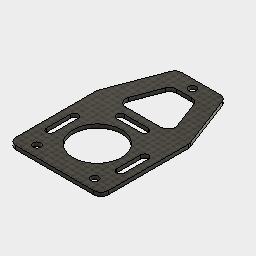
Camera Assembly (Autodesk Fusion 360 archive; units mm, degrees)
design "Camera Mounting Plate"
Autodesk Fusion 360 part; units mm, degrees
sketch "Sketch1" plane through (0, 0, 0) normal (0, 1, 0) x (1, 0, 0)
  circle A0 centre (-12, 0) radius 1.55
  circle A1 centre (12, 0) radius 1.55
  circle A2 centre (0, 13) radius 10
  line L0 (16.1, 13) -> (16.1, 18)
  line L1 (16.1, 13) -> (16.1, 8)
  line L2 (-16.1, 13) -> (-16.1, 18)
  line L3 (-16.1, 13) -> (-16.1, 8)
  line L4 (-13, 13) -> (-13, 18)
  line L5 (-13, 18) -> (-13, 13)
  line L6 (-13, 13) -> (-13, 8)
  line L7 (13, 13) -> (13, 18)
  line L8 (13, 13) -> (13, 8)
  arc A3 (-13, 18) -> (-16.1, 18) centre (-14.55, 18) ccw
  arc A4 (-16.1, 8) -> (-13, 8) centre (-14.55, 8) ccw
  arc A5 (16.1, 18) -> (13, 18) centre (14.55, 18) ccw
  arc A6 (13, 8) -> (16.1, 8) centre (14.55, 8) ccw
  line L9 (0, 29.1) -> (5, 29.1)
  line L10 (0, 29.1) -> (-5, 29.1)
  line L11 (0, 26) -> (5, 26)
  line L12 (5, 26) -> (0, 26)
  line L13 (0, 26) -> (-5, 26)
  arc A7 (-5, 29.1) -> (-5, 26) centre (-5, 27.55) ccw
  arc A8 (5, 26) -> (5, 29.1) centre (5, 27.55) ccw
  line L14 (12, -4.55) -> (16.1, -4.55)
  line L15 (19.1, -1.55) -> (19.1, 13)
  line L16 (-19.1, 13) -> (-19.1, -1.55)
  line L17 (-16.1, -4.55) -> (12, -4.55)
  arc A9 (16.1, -4.55) -> (19.1, -1.55) centre (16.1, -1.55) ccw
  arc A10 (-19.1, -1.55) -> (-16.1, -4.55) centre (-16.1, -1.55) ccw
  circle A11 centre (0, 52.45) radius 1.55
  line L18 (0, 55.95) -> (-7.9306, 55.95)
  line L19 (-19.1, 13) -> (-19.1, 31.4493)
  line L20 (19.1, 13) -> (19.1, 31.4493)
  line L21 (0, 55.95) -> (7.9306, 55.95)
  line L22 (10.735, 54.0156) -> (18.9044, 32.5148)
  line L23 (-10.735, 54.0156) -> (-18.9044, 32.5148)
  line L24 (0, 48.95) -> (3.1021, 48.95)
  line L25 (0, 48.95) -> (-3.1021, 48.95)
  line L26 (7.2626, 32) -> (-7.2626, 32)
  line L27 (10.067, 36.0656) -> (5.9065, 47.0156)
  line L28 (-10.067, 36.0656) -> (-5.9065, 47.0156)
  arc A12 (-10.067, 36.0656) -> (-7.2626, 32) centre (-7.2626, 35) ccw
  arc A13 (7.2626, 32) -> (10.067, 36.0656) centre (7.2626, 35) ccw
  arc A14 (5.9065, 47.0156) -> (3.1021, 48.95) centre (3.1021, 45.95) ccw
  arc A15 (-3.1021, 48.95) -> (-5.9065, 47.0156) centre (-3.1021, 45.95) ccw
  arc A16 (-18.9044, 32.5148) -> (-19.1, 31.4493) centre (-16.1, 31.4493) ccw
  arc A17 (19.1, 31.4493) -> (18.9044, 32.5148) centre (16.1, 31.4493) ccw
  arc A18 (10.735, 54.0156) -> (7.9306, 55.95) centre (7.9306, 52.95) ccw
  arc A19 (-7.9306, 55.95) -> (-10.735, 54.0156) centre (-7.9306, 52.95) ccw
  point P0 (-10, 55.95)
  point P1 (10, 55.95)
extrude "Extrude1" add sketch "Sketch1" along normal blind 1.5

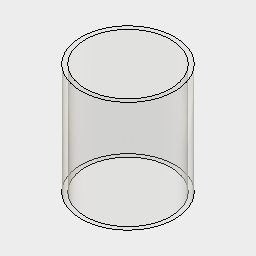
design "Acryllic Tube"
Autodesk Fusion 360 part; units mm, degrees
sketch "Sketch1" plane through (0, 0, 0) normal (0, 1, 0) x (1, 0, 0)
  circle A0 centre (0, 0) radius 27.5
  circle A1 centre (0, 0) radius 25
  dimension "d1" = 55
  measures "d1" diameter of A0
extrude "Extrude1" add sketch "Sketch1" along normal blind 65

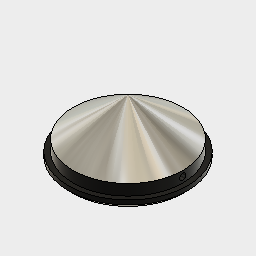
design "Camera Cap"
Autodesk Fusion 360 part; units mm, degrees
sketch "Sketch1" plane through (0, 0, 0) normal (0, 1, 0) x (1, 0, 0)
  circle A0 centre (0, 0) radius 27.5
  dimension "d1" = 55
  measures "d1" diameter of A0
extrude "Extrude1" add sketch "Sketch1" along normal blind 4
sketch "Sketch2" plane through (0, 4, 0) normal (0, 1, 0) x (-1, 0, 0)
  circle A0 centre (0, 0) radius 27.5
  circle A1 centre (0, 0) radius 25.3
  dimension "d4" = 50.6
  measures "d4" diameter of A1
extrude "Extrude2" add sketch "Sketch2" along normal blind 5 contours A1
sketch "Sketch3" plane through (0, 0, 0) normal (0, -1, 0) x (1, 0, 0)
  circle A0 centre (0, 0) radius 27.5
  line L0 (21.5985, 0) -> (19.1914, -4.1689)
  line L1 (3.5784, -14.5357) -> (-13.1761, -14.5877)
  line L2 (-11.9706, 0) -> (-14.3773, 4.1693)
  line L3 (-14.3773, 4.1693) -> (-5.9851, -10.3664)
  line L4 (14.3777, -4.1689) -> (6.0451, -18.7046)
  line L5 (5.9851, -10.3664) -> (3.5784, -14.5357)
  line L6 (-14.3773, 4.1693) -> (-6.0451, 18.705)
  line L7 (-5.9851, 18.705) -> (-14.3773, 4.1693)
  line L8 (-10.7992, -10.3664) -> (-19.2216, 4.1173)
  line L9 (-19.1914, 4.1693) -> (-10.7992, -10.3664)
  line L10 (-10.7992, -18.7046) -> (-13.2063, -14.5357)
  line L11 (-5.9851, -10.3664) -> (-10.7992, -10.3664)
  line L12 (-21.5985, 0) -> (-19.1914, 4.1693)
  line L13 (10.7992, 10.3668) -> (19.2216, -4.1169)
  line L14 (-10.7992, -10.3664) -> (5.9851, -10.3664)
  line L15 (-13.2063, -14.5357) -> (3.5784, -14.5357)
  line L16 (14.3777, -4.1689) -> (5.9851, 10.3668)
  line L17 (13.2063, 14.5357) -> (-3.578, 14.5357)
  line L18 (6.0451, -18.7046) -> (-10.7992, -18.7046)
  line L19 (11.9706, 0) -> (14.3777, -4.1689)
  line L20 (19.1914, -4.1689) -> (10.7992, 10.3668)
  line L21 (5.9851, -18.7046) -> (14.3777, -4.1689)
  line L22 (13.1765, 14.5877) -> (21.5985, 0)
  line L23 (-6.0451, 18.705) -> (10.7992, 18.705)
  line L24 (-3.578, 14.5357) -> (-11.9706, 0)
  line L25 (10.7992, 10.3668) -> (-5.9851, 10.3668)
  line L26 (10.7992, -18.7046) -> (5.9851, -18.7046)
  line L27 (19.2216, -4.1169) -> (10.7992, -18.7046)
  line L28 (10.7992, 18.705) -> (13.2063, 14.5357)
  line L29 (-11.9706, 0) -> (11.9706, 0)
  line L30 (0, 0) -> (0, 10.3668)
  line L31 (-19.2216, 4.1173) -> (-10.7992, 18.705)
  line L32 (-13.1761, -14.5877) -> (-21.5985, 0)
  line L33 (-10.7992, 18.705) -> (-5.9851, 18.705)
  line L34 (3.5784, -14.5357) -> (11.9706, 0)
  line L35 (5.9851, 10.3668) -> (10.7992, 10.3668)
  line L36 (-3.578, 14.5357) -> (13.1765, 14.5877)
  line L37 (-5.9851, 10.3668) -> (-3.578, 14.5357)
  line L38 (-13.2236, 4.171) -> (-5.4656, 17.705)
  line L39 (-5.4656, 17.705) -> (10.2219, 17.705)
  line L40 (10.2219, 17.705) -> (11.4743, 15.5357)
  line L41 (11.4743, 15.5357) -> (-4.1554, 15.5357)
  line L42 (-4.1554, 15.5357) -> (-11.9705, 2.0001)
  line L43 (-11.9705, 2.0001) -> (-13.2236, 4.171)
  line L44 (11.3766, 11.3668) -> (-4.253, 11.3668)
  line L45 (-4.253, 11.3668) -> (-2.9997, 13.5375)
  line L46 (-2.9997, 13.5375) -> (12.6002, 13.5859)
  line L47 (12.6002, 13.5859) -> (20.4438, 0)
  line L48 (20.4438, 0) -> (19.1914, -2.1689)
  line L49 (19.1914, -2.1689) -> (11.3766, 11.3668)
  line L50 (10.224, 9.3668) -> (18.0659, -4.1187)
  line L51 (18.0659, -4.1187) -> (10.2219, -17.7046)
  line L52 (10.2219, -17.7046) -> (7.7172, -17.7046)
  line L53 (7.7172, -17.7046) -> (15.5324, -4.1689)
  line L54 (15.5324, -4.1689) -> (7.7172, 9.3668)
  line L55 (7.7172, 9.3668) -> (10.224, 9.3668)
  line L56 (13.224, -4.1707) -> (5.4657, -17.7046)
  line L57 (5.4657, -17.7046) -> (-10.2219, -17.7046)
  line L58 (-10.2219, -17.7046) -> (-11.4742, -15.5357)
  line L59 (-11.4742, -15.5357) -> (4.1558, -15.5357)
  line L60 (4.1558, -15.5357) -> (11.9706, -2)
  line L61 (11.9706, -2) -> (13.224, -4.1707)
  line L62 (3, -13.5375) -> (-12.5998, -13.5859)
  line L63 (-12.5998, -13.5859) -> (-20.4438, 0)
  line L64 (-20.4438, 0) -> (-19.1914, 2.1693)
  line L65 (-19.1914, 2.1693) -> (-11.3766, -11.3664)
  line L66 (-11.3766, -11.3664) -> (4.2532, -11.3664)
  line L67 (4.2532, -11.3664) -> (3, -13.5375)
  line L68 (-10.224, -9.3664) -> (-18.0659, 4.1191)
  line L69 (-18.0659, 4.1191) -> (-10.2219, 17.705)
  line L70 (-10.2219, 17.705) -> (-7.7172, 17.705)
  line L71 (-7.7172, 17.705) -> (-15.532, 4.1693)
  line L72 (-15.532, 4.1693) -> (-7.7172, -9.3664)
  line L73 (-7.7172, -9.3664) -> (-10.224, -9.3664)
  dimension "d8" = 1
  dimension "d9" = 1
  dimension "d10" = 1
  dimension "d11" = 1
  dimension "d12" = 1
  dimension "d13" = 1
extrude "Extrude3" cut sketch "Sketch3" against normal blind 1 contours L38 L39 L40 L41 L42 L43 | L44 L45 L46 L47 L48 L49 | L50 L51 L52 L53 L54 L55 | L56 L57 L58 L59 L60 L61 | L62 L63 L64 L65 L66 L67 | L68 L69 L70 L71 L72 L73
chamfer "Chamfer1" distance 2 angle 45 1 edges at (-25.639, 0, 9.9444)
sketch "Sketch5" plane through (0, 0, 0) normal (0, 0, 1) x (1, 0, 0)
  line L0 (25.3, 9) -> (-25.3, 9)
  line L1 (25.3, 9) -> (0, 26.7153)
  line L2 (25.3, 9) -> (54.9449, 9) construction
  line L3 (0, 26.7153) -> (0, 9)
  line L4 (0, 26.7153) -> (0, 24.5)
  dimension "d19" = 145
  dimension "d37" = 30.8856
  measures "d19" angle of L1 L2
  measures "d37" distance of L0.start L1.end
revolve "Revolve1" add sketch "Sketch5" angle 360 about axis through (0, 1.75, 0) along (0, 1, 0)
ref_plane "WorkPlane3" through (25.3, 0, 0) normal (1, 0, 0) x (0, 1, 0)
sketch "Sketch8" plane through (25.3, 0, 0) normal (1, 0, 0) x (0, 0, -1)
  line L0 (0, 9) -> (0, 6.5)
  circle A0 centre (0, 6.5) radius 1.4
  point P0 (0, 9)
  dimension "d28" = 2.5
  dimension "d29" = 2.8
  measures "d28" distance of P0 L0.end
  measures "d29" diameter of A0
extrude "Extrude6" cut sketch "Sketch8" against normal blind 8
ref_plane "WorkPlane4" through (-25.3, 0, 0) normal (1, 0, 0) x (0, 1, 0)
sketch "Sketch9" plane through (-25.3, 0, 0) normal (1, 0, 0) x (0, 0, -1)
  line L0 (0, 9) -> (0, 6.5)
  circle A0 centre (0, 6.5) radius 1.4
  point P0 (0, 9)
  dimension "d33" = 2.5
  dimension "d34" = 2.8
  measures "d33" distance of P0 L0.end
  measures "d34" diameter of A0
extrude "Extrude7" cut sketch "Sketch9" along normal blind 8

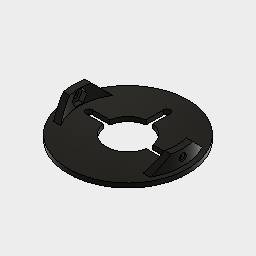
design "Camera Tube Mount"
Autodesk Fusion 360 part; units mm, degrees
sketch "Sketch1" plane through (0, 0, 0) normal (0, 1, 0) x (1, 0, 0)
  circle A0 centre (0, 0) radius 27.5
  circle A1 centre (0, 0) radius 10
  line L0 (0, 0) -> (13, 0)
  line L1 (0, 0) -> (0, 13)
  line L2 (0, 0) -> (-13, 0)
  line L3 (-13, 0) -> (-13, 1.55)
  line L4 (-13, 1.55) -> (-18, 1.55)
  line L5 (-13, 1.55) -> (-9.8791, 1.55)
  line L6 (-13, 0) -> (-13, -1.55)
  line L7 (-13, -1.55) -> (-9.8791, -1.55)
  line L8 (-13, -1.55) -> (-18, -1.55)
  line L9 (0, 13) -> (1.55, 13)
  line L10 (1.55, 13) -> (1.55, 18)
  line L11 (1.55, 18) -> (-1.55, 18)
  line L12 (-1.55, 18) -> (-1.55, 9.8791)
  line L13 (1.55, 9.8791) -> (1.55, 18)
  line L14 (13, 0) -> (13, -1.55)
  line L15 (13, -1.55) -> (18, -1.55)
  line L16 (18, -1.55) -> (9.8791, -1.55)
  line L17 (9.8791, 1.55) -> (18, 1.55)
  line L18 (18, 1.55) -> (18, -1.55)
  arc A2 (-18, 1.55) -> (-18, -1.55) centre (-18, 0) ccw
  arc A3 (1.55, 18) -> (-1.55, 18) centre (0, 18) ccw
  arc A4 (18, -1.55) -> (18, 1.55) centre (18, 0) ccw
  dimension "d12" = 13
  dimension "d13" = 13
  dimension "d14" = 13
  dimension "d15" = 1.55
  dimension "d16" = 5
  dimension "d17" = 1.55
  dimension "d18" = 1.55
  dimension "d19" = 5
  dimension "d20" = 3.1
  dimension "d21" = 1.55
  dimension "d22" = 5
  dimension "d23" = 3.1
  measures "d12" distance of A0.centre L0.end
  measures "d13" distance of A0.centre L1.end
  measures "d14" distance of A0.centre L2.end
  measures "d15" distance of L2.end L3.end
  measures "d16" distance of L3.end L4.end
  measures "d17" distance of L2.end L6.end
  measures "d18" distance of L1.end L9.end
  measures "d19" distance of L9.end L10.end
  measures "d20" distance of L10.end L11.end
  measures "d21" distance of L0.end L14.end
  measures "d22" distance of L14.end L15.end
  measures "d23" distance of L15.end L17.end
extrude "Extrude1" add sketch "Sketch1" along normal blind 2
sketch "Sketch2" plane through (0, 2, 0) normal (0, 1, 0) x (-1, 0, 0)
  line L0 (-18, 1.55) -> (-9.8791, 1.55)
  arc A0 (9.8791, 1.55) -> (-9.8791, 1.55) centre (0, 0) ccw
  line L1 (9.8791, 1.55) -> (18, 1.55)
  arc A1 (18, -1.55) -> (18, 1.55) centre (18, 0) ccw
  line L2 (18, -1.55) -> (9.8791, -1.55)
  arc A2 (1.55, -9.8791) -> (9.8791, -1.55) centre (0, 0) ccw
  line L3 (1.55, -9.8791) -> (1.55, -18)
  arc A3 (-1.55, -18) -> (1.55, -18) centre (0, -18) ccw
  line L4 (-1.55, -18) -> (-1.55, -9.8791)
  arc A4 (-9.8791, -1.55) -> (-1.55, -9.8791) centre (0, 0) ccw
  line L5 (-9.8791, -1.55) -> (-18, -1.55)
  arc A5 (-18, 1.55) -> (-18, -1.55) centre (-18, 0) ccw
  circle A6 centre (0, 0) radius 27.5
  circle A7 centre (0, 0) radius 25.3
  circle A8 centre (0, 0) radius 22.5
  dimension "d26" = 50.6
  dimension "d27" = 45
  measures "d26" diameter of A7
  measures "d27" diameter of A8
extrude "Extrude2" add sketch "Sketch2" along normal blind 7 contours A7
ref_plane "WorkPlane2" through (25.5, 0, 0) normal (1, 0, 0) x (0, 1, 0)
sketch "Sketch4" plane through (25.5, 0, 0) normal (1, 0, 0) x (0, 0, -1)
  line L0 (0, 9) -> (0, 5.5)
  circle A0 centre (0, 5.5) radius 1.6
  point P0 (0, 9)
  dimension "d35" = 3.5
  dimension "d36" = 3.2
  measures "d35" distance of P0 L0.end
  measures "d36" diameter of A0
extrude "Extrude4" cut sketch "Sketch4" against normal through all
ref_plane "WorkPlane3" through (22.5, 0, 0) normal (1, 0, 0) x (0, 1, 0)
sketch "Sketch5" plane through (22.5, 0, 0) normal (1, 0, 0) x (0, 0, -1)
  line L0 (-1.7321, 8.5) -> (-3.4641, 5.5)
  line L1 (-3.4641, 5.5) -> (-1.7321, 2.5)
  line L2 (-1.7321, 2.5) -> (1.7321, 2.5)
  line L3 (1.7321, 2.5) -> (3.4641, 5.5)
  line L4 (3.4641, 5.5) -> (1.7321, 8.5)
  line L5 (1.7321, 8.5) -> (-1.7321, 8.5)
  point P0 (0, 5.5)
extrude "Extrude5" cut sketch "Sketch5" along normal blind 2 and the other way blind 1
pattern_circular "C-Pattern1" count 2 over 360 about axis through (0, 1.75, 0) along (0, 1, 0) of "Extrude5"
sketch "Sketch6" plane through (0, 0, 0) normal (1, 0, 0) x (0, 0, -1)
  line L0 (0, 9) -> (-2, 9)
  line L1 (1.55, 2) -> (9.8791, 2)
  line L2 (27.5, 2) -> (-27.5, 2)
  line L3 (28, 9) -> (28, 2)
  line L4 (28, 2) -> (-25.7716, 2)
  line L5 (-25.7716, 2) -> (-25.7716, 9)
  line L6 (0, 9) -> (-5, 9)
  line L7 (0, 9) -> (5, 9)
  line L8 (5, 9) -> (12, 2)
  line L9 (5, 9) -> (14.8995, 9) construction
  line L10 (-5, 9) -> (-12, 2)
  line L11 (28, 9) -> (-26, 9)
  point P0 (0, 9)
  dimension "d46" = 2
  dimension "d52" = 5
  dimension "d53" = 5
  dimension "d54" = 45
  measures "d46" distance of P0 L0.end
  measures "d52" distance of P0 L6.end
  measures "d53" distance of P0 L7.end
  measures "d54" angle of L8 L9
extrude "Extrude8" cut sketch "Sketch6" along normal mid plane 57.44 contours L2 L3 L4 L8 L11 | L2 L4 L5 L10 L11
